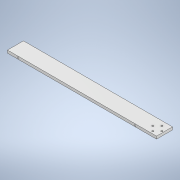
# Autodesk Inventor part: 横長2ndフラットバー
Saved by Autodesk Inventor 2022 (Build 260153000, 153)
## iProperties
Created: 2022-10-17
Part Number: 横長2ndフラットバー
Material: アルミニウム
Document SubType Name: Modeling
Designer: tdn82
Density: 2.7 g/cm^3
Appearance: サテン
Author: tdn82
Autodesk Inventor part; units mm, degrees
ref_plane "YZ Plane" through (0, 0, 0) normal (1, 0, 0) x (0, 1, 0)
ref_plane "XZ Plane" through (0, 0, 0) normal (0, 1, 0) x (-1, 0, 0)
ref_plane "XY Plane" through (0, 0, 0) normal (0, 0, 1) x (1, 0, 0)
sketch "スケッチ1" plane through (0, 0, 0) normal (1, 0, 0) x (0, 1, 0)
  line L0 (0, 0) -> (-5, 0)
  line L1 (-5, 0) -> (-5, -30)
  line L2 (-5, -30) -> (0, -30)
  line L3 (0, -30) -> (0, 0)
  dimension "d0" = 30
  dimension "d1" = 5
  constraints: 8 end point, 2 parallel, 1 horizontal, 1 perpendicular
  measures "d0" distance of L2.end L0.start
  measures "d1" distance of L0.start L0.end
extrude "押し出し1" add sketch "スケッチ1" along normal blind 280
sketch "スケッチ2" plane through (0, -5, -30) normal (0, -1, 0) x (1, 0, 0)
  line L0 (280, 30) -> (280, 0) projected
  line L1 (0, 0) -> (280, 0) projected
  point P0 (0, 30)
  point P1 (268.5, 17)
  dimension "d4" = 11.5
  dimension "d12" = 17
  measures "d4" distance from line of point (268.5, 17) L0
  measures "d12" distance from line of point (268.5, 17) L1
hole "穴1" at (268.5, -5, -13) direction (0, 1, 0) diameter 10 depth 1.5 tip angle 118
sketch "スケッチ4" plane through (280, 0, -30) normal (0, 0, -1) x (-1, 0, 0)
  line L0 (280, 0) -> (0, 0) projected
  line L1 (280, -5) -> (280, 0) projected
  point P0 (260, -2.5)
  point P1 (40, -2.5)
  dimension "d27" = 2.5
  dimension "d28" = 20
  dimension "d36" = 220
  measures "d27" distance from line of point (260, -2.5) L0
  measures "d28" distance from line of point (260, -2.5) L1
  measures "d36" distance of point (40, -2.5) point (260, -2.5)
hole "穴3" at (20, -2.5, -30) at (240, -2.5, -30) direction (0, 0, 1) diameter 2.459 end through all thread size "M3x0.5" class "6H" standard "ANSI Metric M Profile"
sketch "スケッチ5" plane through (0, -5, -30) normal (0, -1, 0) x (1, 0, 0)
  circle A0 centre (268.5, 17) radius 5 projected
  point P0 (0, 30)
  point P1 (268.5, 8.5)
  point P2 (277, 17)
  point P3 (268.5, 25.5)
  point P4 (260, 17)
  dimension "d39" = 360
  dimension "d41" = 8.5
  constraints: 5 other
  measures "d41" distance of point (268.5, 8.5) A0.centre
hole "穴4" at (268.5, -5, -21.5) at (277, -5, -13) at (268.5, -5, -4.5) at (260, -5, -13) direction (0, 1, 0) diameter 3 end through all
